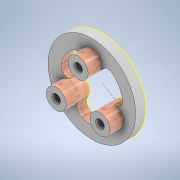
# Autodesk Inventor part: palm_connector
Saved by Autodesk Inventor 2021 (Build 250183000, 183)
## iProperties
Created: 2021-05-31
Part Number: palm_connector
Material: Generic
Document SubType Name: Modeling
Designer: ztjona!
Density: 1 g/cm^3
Appearance: Default
Author: ztjona!
Autodesk Inventor part; units mm, degrees
ref_plane "YZ Plane" through (0, 0, 0) normal (1, 0, 0) x (0, 1, 0)
ref_plane "XZ Plane" through (0, 0, 0) normal (0, 1, 0) x (-1, 0, 0)
ref_plane "XY Plane" through (0, 0, 0) normal (0, 0, 1) x (1, 0, 0)
sketch "Sketch1" plane through (0, 0, 0) normal (0, 0, 1) x (1, 0, 0)
  arc A0 (17.5247, -11.3882) -> (16.1661, 13.211) centre (-0.0131, -0.0197) ccw projected
  arc A1 (16.1661, 13.211) -> (-17.4371, 11.522) centre (-0.0129, -0.0197) ccw projected
  arc A2 (-17.4371, 11.522) -> (17.5247, -11.3882) centre (0.0128, 0.0195) ccw projected
  circle A3 centre (0.0128, 0.0195) radius 16.547 projected
  arc A4 (-0.8003, 20.8657) -> (0.7744, -20.905) centre (-0.0131, -0.0197) ccw projected
  line L0 (-0.8003, 20.8657) -> (-0.868, 22.6615) projected
  line L1 (-0.868, 22.6615) -> (-2.5183, 22.5224) projected
  arc A5 (-2.5183, 22.5224) -> (-2.5534, 22.518) centre (0.1238, 1.0382) ccw projected
  line L2 (-2.5534, 22.518) -> (-4.1105, 22.266) projected
  arc A6 (-4.1105, 22.266) -> (-4.2428, 22.2392) centre (0.1238, 1.0382) ccw projected
  line L3 (-4.2428, 22.2392) -> (-5.6625, 21.8965) projected
  arc A7 (-5.6625, 21.8965) -> (-5.9115, 21.8258) centre (0.1238, 1.0382) ccw projected
  line L4 (-5.9115, 21.8258) -> (-7.1946, 21.4095) projected
  arc A8 (-7.1946, 21.4095) -> (-7.7258, 21.2108) centre (0.1238, 1.0382) ccw projected
  line L5 (-7.7258, 21.2108) -> (-8.9127, 20.7078) projected
  arc A9 (-8.9127, 20.7078) -> (-9.2791, 20.5353) centre (0.1238, 1.0382) ccw projected
  line L6 (-9.2791, 20.5353) -> (-10.3934, 19.9575) projected
  arc A10 (-10.3934, 19.9575) -> (-10.7425, 19.7592) centre (0.1238, 1.0382) ccw projected
  line L7 (-10.7425, 19.7592) -> (-11.8208, 19.0903) projected
  arc A11 (-11.8208, 19.0903) -> (-12.124, 18.8859) centre (0.1238, 1.0382) ccw projected
  line L8 (-12.124, 18.8859) -> (-13.195, 18.1017) projected
  arc A12 (-13.195, 18.1017) -> (-13.9625, 17.4738) centre (0.1238, 1.0382) ccw projected
  line L9 (-13.9625, 17.4738) -> (-15.0896, 16.4363) projected
  arc A13 (-15.0896, 16.4363) -> (-15.145, 16.3815) centre (0.1238, 1.0382) ccw projected
  line L10 (-15.145, 16.3815) -> (-16.2632, 15.1782) projected
  line L11 (-16.2632, 15.1782) -> (-17.3134, 13.8584) projected
  line L12 (-17.3134, 13.8584) -> (-18.2689, 12.4514) projected
  line L13 (-18.2689, 12.4514) -> (-18.5334, 12.0182) projected
  line L14 (-18.5334, 12.0182) -> (-19.3688, 10.4871) projected
  line L15 (-19.3688, 10.4871) -> (-20.083, 8.911) projected
  line L16 (-20.083, 8.911) -> (-20.6779, 7.2958) projected
  line L17 (-20.6779, 7.2958) -> (-21.152, 5.6438) projected
  line L18 (-21.152, 5.6438) -> (-21.5797, 3.4669) projected
  line L19 (-21.5797, 3.4669) -> (-21.7618, 1.7835) projected
  line L20 (-21.7618, 1.7835) -> (-21.8161, 0.1003) projected
  line L21 (-21.8161, 0.1003) -> (-21.7428, -1.583) projected
  line L22 (-21.7428, -1.583) -> (-21.6202, -2.7239) projected
  line L23 (-21.6202, -2.7239) -> (-21.3264, -4.4266) projected
  line L24 (-21.3264, -4.4266) -> (-20.9055, -6.0981) projected
  line L25 (-20.9055, -6.0981) -> (-20.3593, -7.738) projected
  line L26 (-20.3593, -7.738) -> (-19.6908, -9.3414) projected
  line L27 (-19.6908, -9.3414) -> (-18.6931, -11.2832) projected
  line L28 (-18.6931, -11.2832) -> (-17.6782, -12.8711) projected
  line L29 (-17.6782, -12.8711) -> (-16.6668, -14.2237) projected
  line L30 (-16.6668, -14.2237) -> (-15.5609, -15.4938) projected
  line L31 (-15.5609, -15.4938) -> (-14.8459, -16.2211) projected
  line L32 (-14.8459, -16.2211) -> (-13.5887, -17.3523) projected
  line L33 (-13.5887, -17.3523) -> (-12.2623, -18.3753) projected
  line L34 (-12.2623, -18.3753) -> (-10.8699, -19.2905) projected
  line L35 (-10.8699, -19.2905) -> (-9.4133, -20.0965) projected
  arc A14 (-9.4133, -20.0965) -> (-9.4126, -20.0968) centre (0.1074, -0.7797) ccw projected
  line L36 (-9.4126, -20.0968) -> (-8.8344, -20.3712) projected
  arc A15 (-8.8344, -20.3712) -> (0.8271, -22.3033) centre (0.1074, -0.7797) ccw projected
  line L37 (0.8271, -22.3033) -> (0.8159, -22.0051) projected
  line L38 (0.8159, -22.0051) -> (0.7744, -20.905) projected
  line L39 (11.5292, 18.7089) -> (8.9194, 20.0849) projected
  line L40 (8.9194, 20.0849) -> (6.0582, 21.1256) projected
  line L41 (6.0582, 21.1256) -> (3.0061, 21.7717) projected
  line L42 (3.0061, 21.7717) -> (0.1167, 21.9794) projected
  line L43 (0.1167, 21.9794) -> (-0.8418, 21.9647) projected
  line L44 (-0.8003, 20.8657) -> (-0.8418, 21.9647) projected
  arc A16 (16.1661, 13.211) -> (-0.8003, 20.8657) centre (-0.0131, -0.0197) ccw projected
  arc A17 (6.9882, -19.7123) -> (16.1661, 13.211) centre (-0.0129, -0.0197) ccw projected
  arc A18 (0.7744, -20.905) -> (6.9882, -19.7123) centre (-0.0131, -0.0197) ccw projected
  line L45 (0.8159, -22.0051) -> (0.7744, -20.905) projected
  line L46 (0.8159, -22.0051) -> (3.8656, -21.6756) projected
  line L47 (3.8656, -21.6756) -> (6.8541, -20.921) projected
  line L48 (6.8541, -20.921) -> (9.7319, -19.7442) projected
  line L49 (9.7319, -19.7442) -> (12.4411, -18.1557) projected
  line L50 (12.4411, -18.1557) -> (14.8907, -16.2028) projected
  line L51 (14.8907, -16.2028) -> (16.5899, -14.4545) projected
  line L52 (16.5899, -14.4545) -> (18.4499, -11.9835) projected
  line L53 (18.4499, -11.9835) -> (19.9467, -9.2727) projected
  line L54 (19.9467, -9.2727) -> (21.0432, -6.3956) projected
  line L55 (21.0432, -6.3956) -> (21.7254, -3.4018) projected
  line L56 (21.7254, -3.4018) -> (21.9848, -0.332) projected
  line L57 (21.9848, -0.332) -> (21.9404, 1.4116) projected
  line L58 (21.9404, 1.4116) -> (21.5354, 4.4148) projected
  line L59 (21.5354, 4.4148) -> (20.7192, 7.3405) projected
  line L60 (20.7192, 7.3405) -> (19.5101, 10.1214) projected
  line L61 (19.5101, 10.1214) -> (17.9894, 12.6256) projected
  line L62 (17.9894, 12.6256) -> (16.1099, 14.9483) projected
  line L63 (16.1099, 14.9483) -> (13.8991, 17.0226) projected
  line L64 (13.8991, 17.0226) -> (11.5292, 18.7089) projected
  line L65 (-8.7456, -2.1504) -> (-11.2456, -3.5937)
  line L66 (-11.2456, -3.5937) -> (-11.2456, -6.4805)
  line L67 (-11.2456, -6.4805) -> (-8.7456, -7.9239)
  line L68 (-8.7456, -7.9239) -> (-6.2456, -6.4805)
  line L69 (-6.2456, -6.4805) -> (-6.2456, -3.5937)
  line L70 (-6.2456, -3.5937) -> (-8.7456, -2.1504)
  circle A19 centre (-8.7456, -5.0371) radius 4
  line L71 (-6.2456, -5.0371) -> (-11.2456, -5.0371) construction
  line L72 (-8.7456, -2.1504) -> (-8.7456, -5.0371) construction
  circle A20 centre (0.0128, 0.0195) radius 14.5 construction
  line L73 (-12.5446, -7.2305) -> (0.0128, 14.5195) construction
  line L74 (0.0128, 14.5195) -> (12.5701, -7.2305) construction
  line L75 (12.5701, -7.2305) -> (-12.5446, -7.2305) construction
  line L76 (0.0128, 0.0195) -> (-11.2456, -6.4805) construction
  line L77 (0.0128, 0.0195) -> (0.0128, 14.5195) construction
  line L78 (12.5701, -7.2305) -> (0.0128, 0.0195) construction
  line L79 (-11.2456, -6.4805) -> (-12.5446, -7.2305)
  circle A21 centre (0.0128, 10.1328) radius 4
  line L80 (2.5128, 11.5761) -> (0.0128, 13.0195)
  line L81 (2.5128, 8.6894) -> (2.5128, 11.5761)
  line L82 (0.0128, 7.246) -> (2.5128, 8.6894)
  line L83 (-2.4872, 8.6894) -> (0.0128, 7.246)
  line L84 (-2.4872, 11.5761) -> (-2.4872, 8.6894)
  line L85 (0.0128, 13.0195) -> (-2.4872, 11.5761)
  circle A22 centre (8.7711, -5.0371) radius 4
  line L86 (8.7711, -7.9239) -> (11.2711, -6.4805)
  line L87 (6.2711, -6.4805) -> (8.7711, -7.9239)
  line L88 (6.2711, -3.5937) -> (6.2711, -6.4805)
  line L89 (8.7711, -2.1504) -> (6.2711, -3.5937)
  line L90 (11.2711, -3.5937) -> (8.7711, -2.1504)
  line L91 (11.2711, -6.4805) -> (11.2711, -3.5937)
  circle A23 centre (0.0128, 0.0195) radius 12.5
  circle A24 centre (0.0128, 0.0195) radius 17.5
  point P0 (0, 0)
  point P1 (0, 0)
  point P2 (1.2628, 12.2978)
  point P3 (-1.2372, 7.9677)
  point P4 (10.0211, -7.2022)
  point P5 (7.5211, -2.872)
  point P6 (-8.6054, -9.0346)
  point P7 (-12.1374, -2.9169)
  point P8 (-3.5193, 12.0101)
  point P9 (3.5448, 12.0101)
  point P10 (12.163, -2.9169)
  point P11 (8.6309, -9.0346)
  point P12 (-10.3201, -7.0148)
  point P13 (-11.2456, -5.4119)
  point P14 (10.3457, -7.0148)
  point P15 (11.2711, -5.4119)
  point P16 (-0.9127, 12.4852)
  point P17 (0.9382, 12.4852)
  point P18 (-11.8438, -3.9391)
  point P19 (-9.3438, -8.2693)
  point P20 (9.3694, -8.2693)
  point P21 (11.8694, -3.9391)
  point P22 (2.5128, 12.267)
  point P23 (-2.4872, 12.267)
  dimension "d12" = 5
  dimension "d13" = 8
  dimension "d14" = 5
  dimension "d15" = 1.5
  dimension "d16" = 360
  dimension "d18" = 25
  dimension "d22" = 3
  dimension "d28" = 2
  constraints: 54 end point, 5 centre point, 3 equal length, 3 midpoint, 2 coincident, 2 horizontal, 2 parallel, 2 vertical, 1 perpendicular, 1 point on line, 60 other
  measures "d12" distance between parallel lines of L69 L66
  measures "d13" diameter of A19
  measures "d14" distance between parallel lines of L65 L68
  measures "d15" distance of L76.end L73.start
  measures "d18" diameter of A23
extrude "Extrusion2" add sketch "Sketch1" along normal blind 4 contours A3 | L65 L66 A23 A19 L67 L68 L69 L70 | L66 L79 A19 A23 | L67 A23 A19 L79 | A23 L85 L84 L83 L82 L81 L80 A21 | A21 A23 L80 L85 | A23 L86 L91 A22 | A22 A23 L91 L90 L89 L88 L87 L86 | A24
sketch "Sketch3" plane through (0.0128, 0.0195, 4) normal (0, 0, 1) x (1, 0, 0)
  arc A0 (-3.5321, 11.9906) -> (3.5321, 11.9906) centre (0, 10.1132) ccw projected
  arc A1 (12.1502, -2.9364) -> (3.5321, 11.9906) centre (0, 0) ccw projected
  arc A2 (12.1502, -2.9364) -> (8.6181, -9.0542) centre (8.7583, -5.0566) ccw projected
  arc A3 (-8.6181, -9.0542) -> (8.6181, -9.0542) centre (0, 0) ccw projected
  arc A4 (-8.6181, -9.0542) -> (-12.1502, -2.9364) centre (-8.7583, -5.0566) ccw projected
  arc A5 (-3.5321, 11.9906) -> (-12.1502, -2.9364) centre (0, 0) ccw projected
  line L0 (0, 7.2265) -> (-2.5, 8.6699) projected
  line L1 (-2.5, 8.6699) -> (-2.5, 11.5566) projected
  line L2 (-2.5, 11.5566) -> (0, 13) projected
  line L3 (0, 13) -> (2.5, 11.5566) projected
  line L4 (2.5, 11.5566) -> (2.5, 8.6699) projected
  line L5 (2.5, 8.6699) -> (0, 7.2265) projected
  circle A6 centre (0, 0) radius 17.5 projected
  line L6 (8.7583, -2.1699) -> (11.2583, -3.6132) projected
  line L7 (11.2583, -3.6132) -> (11.2583, -6.5) projected
  line L8 (11.2583, -6.5) -> (8.7583, -7.9434) projected
  line L9 (8.7583, -7.9434) -> (6.2583, -6.5) projected
  line L10 (6.2583, -6.5) -> (6.2583, -3.6132) projected
  line L11 (6.2583, -3.6132) -> (8.7583, -2.1699) projected
  line L12 (-11.2583, -6.5) -> (-11.2583, -3.6132) projected
  line L13 (-11.2583, -3.6132) -> (-8.7583, -2.1699) projected
  line L14 (-8.7583, -2.1699) -> (-6.2583, -3.6132) projected
  line L15 (-6.2583, -3.6132) -> (-6.2583, -6.5) projected
  line L16 (-6.2583, -6.5) -> (-8.7583, -7.9434) projected
  line L17 (-8.7583, -7.9434) -> (-11.2583, -6.5) projected
  circle A7 centre (-8.7583, -5.0566) radius 1.5
  circle A8 centre (0, 10.1132) radius 1.5
  circle A9 centre (8.7583, -5.0566) radius 1.5
  circle A10 centre (-8.7583, -5.0566) radius 4
  circle A11 centre (8.7583, -5.0566) radius 4
  arc A12 (-3.5321, 11.9906) -> (3.5321, 11.9906) centre (0, 10.1132) ccw projected
  arc A13 (12.1502, -2.9364) -> (8.6181, -9.0542) centre (8.7583, -5.0566) ccw projected
  circle A14 centre (0, 10.1132) radius 4
  point P0 (-0.0128, -0.0195)
  point P1 (3.9284, 11.8667)
  point P2 (-3.9284, 11.8667)
  point P3 (-12.1502, -2.9364)
  point P4 (-8.6181, -9.0542)
  point P5 (12.241, -2.5312)
  point P6 (8.3126, -9.3354)
  point P7 (3.7826, 11.9139)
  point P8 (-3.5321, 11.9906)
  point P9 (-3.5321, 11.9906)
  point P10 (-12.241, -2.5312)
  point P11 (-4.7583, -5.0566)
  point P12 (8.4265, -9.2328)
  point P13 (12.2091, -2.6811)
  point P14 (4, 10.1132)
  point P15 (-3.7826, 11.9139)
  point P16 (-12.2091, -2.6811)
  point P17 (-12.1502, -2.9364)
  point P18 (-8.6181, -9.0542)
  point P19 (-8.4265, -9.2328)
  point P20 (-3.5321, 11.9906)
  point P21 (-6.9787, -8.639)
  point P22 (-10.9709, -1.7243)
  dimension "d16" = 360
  dimension "d23" = 3
  dimension "d24" = 3
  dimension "d25" = 3
  constraints: 6 centre point, 5 coincident, 4 concentric
  measures "d23" diameter of A7
  measures "d24" diameter of A8
  measures "d25" diameter of A9
extrude "Extrusion3" [suppressed]
fillet "Fillet1" radius 3 6 edges at (-12.1374, -2.9169, 2) (-8.6054, -9.0346, 2) (3.5448, 12.0101, 2) (12.163, -2.9169, 2) (8.6309, -9.0346, 2) (-3.5193, 12.0101, 2)
sketch "Boceto4" plane through (0.0128, 0.0195, 0) normal (0, 0, -1) x (-1, 0, 0)
  arc A0 (-3.6093, 8.3891) -> (-8.311, 9.3369) centre (-6.3164, 7.096) ccw projected
  arc A1 (-3.6093, 8.3891) -> (3.6093, 8.3891) centre (0, 10.1132) ccw projected
  arc A2 (8.311, 9.3369) -> (3.6093, 8.3891) centre (6.3164, 7.096) ccw projected
  arc A3 (12.2415, 2.5291) -> (8.311, 9.3369) centre (0, 0) ccw projected
  arc A4 (9.0699, -1.0688) -> (12.2415, 2.5291) centre (9.3035, 1.9221) ccw projected
  arc A5 (9.0699, -1.0688) -> (5.4605, -7.3203) centre (8.7583, -5.0566) ccw projected
  arc A6 (3.9305, -11.866) -> (5.4605, -7.3203) centre (2.9872, -9.0181) ccw projected
  arc A7 (-3.9305, -11.866) -> (3.9305, -11.866) centre (0, 0) ccw projected
  arc A8 (-5.4605, -7.3203) -> (-3.9305, -11.866) centre (-2.9872, -9.0181) ccw projected
  arc A9 (-5.4605, -7.3203) -> (-9.0699, -1.0688) centre (-8.7583, -5.0566) ccw projected
  arc A10 (-12.2415, 2.5291) -> (-9.0699, -1.0688) centre (-9.3035, 1.9221) ccw projected
  arc A11 (-8.311, 9.3369) -> (-12.2415, 2.5291) centre (0, 0) ccw projected
  line L0 (-11.2583, -6.5) -> (-8.7583, -7.9434) projected
  line L1 (-11.2583, -3.6132) -> (-11.2583, -6.5) projected
  line L2 (-8.7583, -2.1699) -> (-11.2583, -3.6132) projected
  line L3 (-6.2583, -3.6132) -> (-8.7583, -2.1699) projected
  line L4 (-6.2583, -6.5) -> (-6.2583, -3.6132) projected
  line L5 (-8.7583, -7.9434) -> (-6.2583, -6.5) projected
  line L6 (11.2583, -6.5) -> (11.2583, -3.6132) projected
  line L7 (8.7583, -7.9434) -> (11.2583, -6.5) projected
  line L8 (6.2583, -6.5) -> (8.7583, -7.9434) projected
  line L9 (6.2583, -3.6132) -> (6.2583, -6.5) projected
  line L10 (8.7583, -2.1699) -> (6.2583, -3.6132) projected
  line L11 (11.2583, -3.6132) -> (8.7583, -2.1699) projected
  circle A12 centre (0, 0) radius 17.5 projected
  line L12 (0, 13) -> (-2.5, 11.5566) projected
  line L13 (2.5, 11.5566) -> (0, 13) projected
  line L14 (2.5, 8.6699) -> (2.5, 11.5566) projected
  line L15 (0, 7.2265) -> (2.5, 8.6699) projected
  line L16 (-2.5, 8.6699) -> (0, 7.2265) projected
  line L17 (-2.5, 11.5566) -> (-2.5, 8.6699) projected
  line L18 (-11.2583, -6.5) -> (0, 0) construction
  point P0 (0.0128, -0.0195)
  constraints: 2 end point
sketch "Sketch5" plane through (0.0128, 0.0195, 4) normal (0, 0, 1) x (1, 0, 0)
  arc A0 (12.2415, 2.5291) -> (8.311, 9.3369) centre (0, 0) ccw projected
  arc A1 (9.0699, -1.0688) -> (12.2415, 2.5291) centre (9.3035, 1.9221) ccw projected
  arc A2 (9.0699, -1.0688) -> (5.4605, -7.3203) centre (8.7583, -5.0566) ccw projected
  arc A3 (3.9305, -11.866) -> (5.4605, -7.3203) centre (2.9872, -9.0181) ccw projected
  arc A4 (-3.9305, -11.866) -> (3.9305, -11.866) centre (0, 0) ccw projected
  arc A5 (-5.4605, -7.3203) -> (-3.9305, -11.866) centre (-2.9872, -9.0181) ccw projected
  arc A6 (-5.4605, -7.3203) -> (-9.0699, -1.0688) centre (-8.7583, -5.0566) ccw projected
  arc A7 (-12.2415, 2.5291) -> (-9.0699, -1.0688) centre (-9.3035, 1.9221) ccw projected
  arc A8 (-8.311, 9.3369) -> (-12.2415, 2.5291) centre (0, 0) ccw projected
  arc A9 (-3.6093, 8.3891) -> (-8.311, 9.3369) centre (-6.3164, 7.096) ccw projected
  arc A10 (-3.6093, 8.3891) -> (3.6093, 8.3891) centre (0, 10.1132) ccw projected
  arc A11 (8.311, 9.3369) -> (3.6093, 8.3891) centre (6.3164, 7.096) ccw projected
  line L0 (11.2583, -6.5) -> (8.7583, -7.9434) projected
  line L1 (8.7583, -7.9434) -> (6.2583, -6.5) projected
  line L2 (6.2583, -6.5) -> (6.2583, -3.6132) projected
  line L3 (6.2583, -3.6132) -> (8.7583, -2.1699) projected
  line L4 (8.7583, -2.1699) -> (11.2583, -3.6132) projected
  line L5 (11.2583, -3.6132) -> (11.2583, -6.5) projected
  line L6 (-11.2583, -6.5) -> (-11.2583, -3.6132) projected
  line L7 (-11.2583, -3.6132) -> (-8.7583, -2.1699) projected
  line L8 (-8.7583, -2.1699) -> (-6.2583, -3.6132) projected
  line L9 (-6.2583, -3.6132) -> (-6.2583, -6.5) projected
  line L10 (-6.2583, -6.5) -> (-8.7583, -7.9434) projected
  line L11 (-8.7583, -7.9434) -> (-11.2583, -6.5) projected
  circle A12 centre (0, 0) radius 17.5 projected
  line L12 (0, 13) -> (2.5, 11.5566) projected
  line L13 (2.5, 11.5566) -> (2.5, 8.6699) projected
  line L14 (2.5, 8.6699) -> (0, 7.2265) projected
  line L15 (0, 7.2265) -> (-2.5, 8.6699) projected
  line L16 (-2.5, 8.6699) -> (-2.5, 11.5566) projected
  line L17 (-2.5, 11.5566) -> (0, 13) projected
  circle A13 centre (-8.7583, -5.0566) radius 4
  circle A14 centre (8.7583, -5.0566) radius 4
  circle A15 centre (0, 10.1132) radius 4
  point P0 (-0.0128, -0.0195)
  point P1 (5.4605, -7.3203)
  point P2 (9.0699, -1.0688)
  point P3 (3.6093, 8.3891)
  point P4 (-3.6093, 8.3891)
  point P5 (-9.0699, -1.0688)
  constraints: 3 centre point, 3 coincident, 3 equal radius
extrude "Extrusion5" add sketch "Sketch5" along normal blind 4 contours A14 A2 | A10 A15 | A13 A6
sketch "Sketch6" plane through (-8.7456, -5.0371, 8) normal (0, 0, 1) x (1, 0, 0)
  circle A0 centre (0, 0) radius 4 projected
  line L0 (-2.5, -1.4434) -> (-2.5, 1.4434) projected
  line L1 (-2.5, 1.4434) -> (0, 2.8868) projected
  line L2 (0, 2.8868) -> (2.5, 1.4434) projected
  line L3 (2.5, 1.4434) -> (2.5, -1.4434) projected
  line L4 (2.5, -1.4434) -> (0, -2.8868) projected
  line L5 (0, -2.8868) -> (-2.5, -1.4434) projected
  circle A1 centre (17.5167, 0) radius 4 projected
  circle A2 centre (17.5167, 0) radius 4 projected
  line L6 (20.0167, -1.4434) -> (17.5167, -2.8868) projected
  line L7 (17.5167, -2.8868) -> (15.0167, -1.4434) projected
  line L8 (15.0167, -1.4434) -> (15.0167, 1.4434) projected
  line L9 (15.0167, 1.4434) -> (17.5167, 2.8868) projected
  line L10 (17.5167, 2.8868) -> (20.0167, 1.4434) projected
  line L11 (20.0167, 1.4434) -> (20.0167, -1.4434) projected
  circle A3 centre (8.7583, 15.1699) radius 4 projected
  line L12 (8.7583, 18.0566) -> (11.2583, 16.6132) projected
  line L13 (11.2583, 16.6132) -> (11.2583, 13.7265) projected
  line L14 (11.2583, 13.7265) -> (8.7583, 12.2831) projected
  line L15 (8.7583, 12.2831) -> (6.2583, 13.7265) projected
  line L16 (6.2583, 13.7265) -> (6.2583, 16.6132) projected
  line L17 (6.2583, 16.6132) -> (8.7583, 18.0566) projected
  circle A4 centre (0, 0) radius 1.75
  circle A5 centre (17.5167, 0) radius 1.75
  circle A6 centre (8.7583, 15.1699) radius 1.75
  point P0 (8.7456, 5.0371)
  dimension "d34" = 3.5
  dimension "d35" = 3.5
  dimension "d36" = 3.5
  constraints: 3 centre point, 2 coincident, 1 concentric
  measures "d34" diameter of A4
  measures "d35" diameter of A5
  measures "d36" diameter of A6
extrude "Extrusion6" add sketch "Sketch6" along normal blind 1.5 contours A0 | L0 L1 L2 L3 L4 L5 | A1 | L6 L7 L8 L9 L10 L11 | A3 | L12 L13 L14 L15 L16 L17
body "Solid2"
